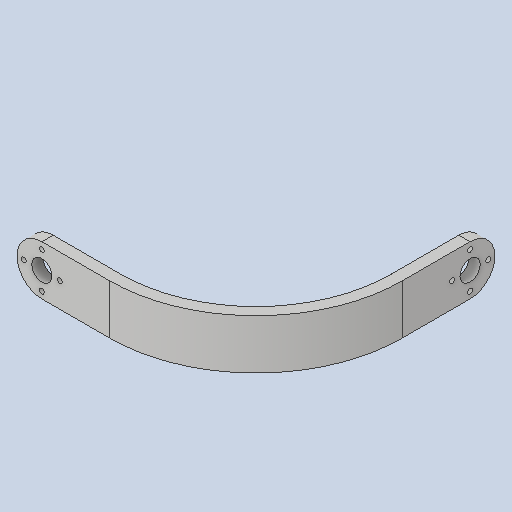
# Autodesk Inventor part: shoulder2
Saved by Autodesk Inventor 2025.1 (Build 291241000, 241)
## iProperties
Created: 2018-10-23
Part Number: shoulder2
Material: 일반
Document SubType Name: Modeling
Designer: otm09
Density: 1 g/cm^3
Appearance: 기본값
Author: otm09
Autodesk Inventor part; units mm, degrees
ref_plane "YZ Plane" through (0, 0, 0) normal (1, 0, 0) x (0, 1, 0)
ref_plane "XZ Plane" through (0, 0, 0) normal (0, 1, 0) x (-1, 0, 0)
ref_plane "XY Plane" through (0, 0, 0) normal (0, 0, 1) x (1, 0, 0)
sketch "스케치1" plane through (0, 0, 0) normal (0, 0, 1) x (1, 0, 0)
  circle A0 centre (0, 0) radius 11
  circle A1 centre (0, -8) radius 1.1
  circle A2 centre (0, 0) radius 11
  circle A3 centre (8, 0) radius 1.1
  circle A4 centre (0, 0) radius 11
  circle A5 centre (0, 8) radius 1.1
  circle A6 centre (0, 0) radius 11
  circle A7 centre (-8, 0) radius 1.1
  arc A8 (-11, 0) -> (11, 0) centre (0, 0) ccw
  circle A9 centre (0, 0) radius 4.5
  line L0 (0, 11) -> (30, 11)
  line L1 (30, 11) -> (30, -11)
  line L2 (30, -11) -> (0, -11)
  arc A10 (0, -11) -> (0, 11) centre (0, 0) ccw
  dimension "d2" = 2.2
  dimension "d3" = 360
  dimension "d4" = 9
  dimension "d5" = 30
  constraints: 11 centre point, 6 end point, 6 point on circle, 4 coincident, 1 horizontal, 1 parallel, 1 perpendicular, 17 other
  measures "d2" diameter of A1
  measures "d4" diameter of A9
  measures "d5" distance of L1.end L2.end
extrude "돌출1" add sketch "스케치1" along normal blind 5
sketch "스케치8" plane through (0, -11, 0) normal (0, -1, 0) x (1, 0, 0)
  line L0 (30, 0) -> (0, 0) projected
  arc A0 (70, -40) -> (30, 0) centre (30, -40) ccw
  line L1 (30, -40) -> (70, -40) construction
  line L2 (30, -40) -> (30, 0) construction
  arc A1 (90, -60) -> (30, 0) centre (30, -60) ccw
  line L3 (30, -60) -> (90, -60) construction
  line L4 (30, -60) -> (30, 0) construction
  dimension "d13" = 90
  dimension "d29" = 90
  constraints: 8 end point, 5 point on circle, 2 centre point
  measures "d13" angle of L1 L2
  measures "d29" angle of L3 L4
sketch "스케치7" plane through (30, -11, 0) normal (1, 0, 0) x (0, 0, -1)
  line L0 (0, 0) -> (-5, 0) projected
  line L1 (0, 22) -> (-5, 22) projected
  line L2 (0, 0) -> (-5, 0)
  line L3 (-5, 0) -> (-5, 22)
  line L4 (-5, 22) -> (0, 22)
  line L5 (0, 22) -> (0, 0)
  point P0 (0, 11)
  constraints: 8 end point, 2 parallel, 1 horizontal, 1 perpendicular
sweep "스윕2" add profiles "스케치7" path "스케치8" path curves A1
sketch "스케치9" plane through (75, -11, -60) normal (0, 0, -1) x (-1, 0, 0)
  line L0 (45, 0) -> (5, 0) projected
  line L1 (5, 22) -> (0, 22) projected
  line L2 (-14.9739, 0) -> (-19.9739, 0)
  line L3 (-19.9739, 0) -> (-19.9739, 22)
  line L4 (-19.9739, 22) -> (-14.9739, 22)
  line L5 (-14.9739, 22) -> (-14.9739, 0)
  point P0 (75, 11)
  constraints: 8 end point, 2 parallel, 1 horizontal, 1 perpendicular
extrude "돌출3" add sketch "스케치9" along normal blind 30
sketch "스케치10" plane through (94.9739, -11, -40) normal (1, 0, 0) x (0, 0, -1)
  line L0 (50, 0) -> (50, 22) projected
  circle A0 centre (50, 11) radius 11
  circle A1 centre (50, 11) radius 4.5
  circle A2 centre (50, 3) radius 1.1
  circle A3 centre (58, 11) radius 1.1
  circle A4 centre (50, 19) radius 1.1
  circle A5 centre (42, 11) radius 1.1
  point P0 (-40, 11)
  dimension "d18" = 9
  dimension "d19" = 2.2
  dimension "d20" = 8
  dimension "d23" = 360
  constraints: 5 centre point, 1 coincident, 1 midpoint, 1 point on line, 1 vertical alignment, 11 other
  measures "d18" diameter of A1
  measures "d19" diameter of A2
  measures "d20" distance of point (50, 11) A2.centre
extrude "돌출4" add sketch "스케치10" against normal blind 5 contours A0 L0 A4 A1 A2 | L0 A2 A1 A4 A0
extrude "돌출5" cut sketch "스케치10" against normal blind 5 contours A2 L0 | L0 A2 | A4 L0 | L0 A4 | A1 L0 | L0 A1 | A5
sketch "스케치11" plane through (89.9739, -11, -60) normal (-1, 0, 0) x (0, 0, 1)
  circle A0 centre (-30, 3) radius 1.1 projected
  circle A1 centre (-30, 3) radius 2.1
  circle A2 centre (-22, 11) radius 1.1 projected
  circle A3 centre (-22, 11) radius 2.1
  circle A4 centre (-38, 11) radius 1.1 projected
  circle A5 centre (-38, 11) radius 2.1
  circle A6 centre (-30, 19) radius 1.1 projected
  circle A7 centre (-30, 19) radius 2.1
  point P0 (60, 11)
  dimension "d30" = 4.2
  dimension "d31" = 4.2
  dimension "d32" = 4.2
  dimension "d33" = 4.2
  constraints: 4 centre point, 4 coincident
  measures "d30" diameter of A1
  measures "d31" diameter of A3
  measures "d32" diameter of A5
  measures "d33" diameter of A7
sketch "스케치12" plane through (0, 0, 0) normal (0, 0, -1) x (-1, 0, 0)
  circle A0 centre (0, -8) radius 1.1 projected
  circle A1 centre (0, -8) radius 2.1
  circle A2 centre (8, 0) radius 1.1 projected
  circle A3 centre (8, 0) radius 2.1
  circle A4 centre (-8, 0) radius 1.1 projected
  circle A5 centre (-8, 0) radius 2.1
  circle A6 centre (0, 8) radius 1.1 projected
  circle A7 centre (0, 8) radius 2.1
  point P0 (0, 0)
  dimension "d34" = 4.2
  dimension "d35" = 4.2
  dimension "d36" = 4.2
  dimension "d37" = 4.2
  constraints: 4 centre point, 4 coincident
  measures "d34" diameter of A1
  measures "d35" diameter of A3
  measures "d36" diameter of A5
  measures "d37" diameter of A7
extrude "돌출6" cut sketch "스케치11" against normal blind 3
extrude "돌출7" cut sketch "스케치12" against normal blind 3
